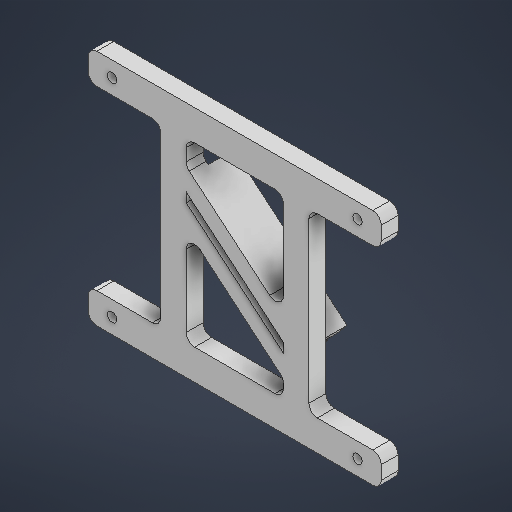
# Autodesk Inventor part: rpi-mount
Saved by Autodesk Inventor 2025 (Build 290162000, 162)
## iProperties
Created: 2024-09-27
Part Number: rpi-mount
Material: Generic
Document SubType Name: Modeling
Designer: Windows 7 was better
Density: 1 g/cm^3
Appearance: Default
Author: Windows 7 was better
Autodesk Inventor part; units mm, degrees
ref_plane "YZ Plane" through (0, 0, 0) normal (1, 0, 0) x (0, 1, 0)
ref_plane "XZ Plane" through (0, 0, 0) normal (0, 1, 0) x (-1, 0, 0)
ref_plane "XY Plane" through (0, 0, 0) normal (0, 0, 1) x (1, 0, 0)
sketch "Sketch1" plane through (0, 0, 0) normal (0, 0, 1) x (1, 0, 0)
  line L0 (35, 0) -> (35, -4)
  line L1 (0, -4) -> (0, 0)
  line L2 (0, 0) -> (0, 1.8) construction
  line L3 (35, 1.8) -> (35, 5.8)
  line L4 (0, 5.8) -> (0, 1.8)
  line L5 (-11.5, 0.9) -> (-11.5, 25.4) construction
  line L6 (-11.5, 25.4) -> (-11.5, -23.6) construction
  line L7 (-11.5, -23.6) -> (46.5, -23.6) construction
  line L8 (-11.5, 25.4) -> (46.5, 25.4) construction
  circle A0 centre (46.5, 25.4) radius 1.1
  circle A1 centre (-11.5, 25.4) radius 1.1
  circle A2 centre (-11.5, -23.6) radius 1.1
  circle A3 centre (46.5, -23.6) radius 1.1
  line L9 (-17.1, -20) -> (52.1, -20)
  line L10 (52.1, -20) -> (52.1, -27.2)
  line L11 (52.1, -27.2) -> (-17.1, -27.2)
  line L12 (-17.1, -27.2) -> (-17.1, -20)
  line L13 (-17.1, -20) -> (52.1, -27.2) construction
  line L14 (52.1, -20) -> (-17.1, -27.2) construction
  line L15 (-17.1, 29) -> (52.1, 29)
  line L16 (52.1, 29) -> (52.1, 21.8)
  line L17 (52.1, 21.8) -> (-17.1, 21.8)
  line L18 (-17.1, 21.8) -> (-17.1, 29)
  line L19 (-17.1, 29) -> (52.1, 21.8) construction
  line L20 (52.1, 29) -> (-17.1, 21.8) construction
  line L21 (35, 21.8) -> (29, 21.8)
  line L22 (29, 21.8) -> (29, -20)
  line L23 (29, -20) -> (35, -20)
  line L24 (35, -20) -> (35, 21.8)
  line L25 (0, 21.8) -> (6, 21.8)
  line L26 (6, 21.8) -> (6, -20)
  line L27 (6, -20) -> (0, -20)
  line L28 (0, -20) -> (0, 21.8)
  line L29 (17.5, 25.4) -> (17.5, 0) construction
  line L30 (17.5, 0) -> (4.0942, 11.2488) construction
  line L31 (4.0942, 11.2488) -> (4.6406, 11.8999) construction
  line L32 (4.6406, 11.8999) -> (3.5479, 10.5976) construction
  line L33 (3.5479, 10.5976) -> (30.3594, -11.8999)
  line L34 (30.3594, -11.8999) -> (27.7883, -14.9641)
  line L35 (27.7883, -14.9641) -> (0.9767, 7.5335)
  line L36 (0.9767, 7.5335) -> (3.5479, 10.5976)
  line L37 (4.6406, 11.8999) -> (31.4521, -10.5976)
  line L38 (31.4521, -10.5976) -> (34.0233, -7.5335)
  line L39 (34.0233, -7.5335) -> (7.2117, 14.9641)
  line L40 (7.2117, 14.9641) -> (4.6406, 11.8999)
  line L41 (27.7883, -14.9641) -> (29, -15.9809)
  line L42 (7.2117, 14.9641) -> (6, 15.9809)
  point P0 (17.5, -23.6)
  point P1 (6, 21.8)
  point P2 (29, 21.8)
  point P3 (0, -20)
  point P4 (35, -20)
  point P5 (29, -3.3184)
  point P6 (6, 13.52)
  point P7 (29, -8.54)
  point P8 (29, -10.7592)
  point P9 (6, 8.54)
  point P10 (6, 10.7592)
  point P11 (29, -13.52)
  point P12 (6, 3.3184)
  dimension "d7" = 24.5
  dimension "d8" = 49
  dimension "d9" = 58
  dimension "d10" = 58
  dimension "d11" = 2.2
  dimension "d12" = 2.2
  dimension "d13" = 2.2
  dimension "d14" = 2.2
  dimension "d15" = 69.2
  dimension "d16" = 7.2
  dimension "d17" = 69.2
  dimension "d18" = 7.2
  dimension "d19" = 6
  dimension "d20" = 6
  dimension "d26" = 17.5
  dimension "d27" = 50
  dimension "d28" = 0.85
  dimension "d29" = 1.7
  dimension "d30" = 35
  dimension "d31" = 4
  dimension "d32" = 4
  constraints: 86 end point, 15 parallel, 9 perpendicular, 9 point on line, 6 horizontal, 6 midpoint, 4 centre point, 4 coincident, 3 vertical
  measures "d7" distance of L5.start L5.end
  measures "d8" distance of L5.end L6.end
  measures "d9" distance of L6.end L7.end
  measures "d10" distance of L5.end L8.end
  measures "d11" diameter of A0
  measures "d12" diameter of A1
  measures "d13" diameter of A2
  measures "d14" diameter of A3
  measures "d15" distance of L10.end L11.end
  measures "d16" distance of L9.end L10.end
  measures "d17" distance of L16.end L17.end
  measures "d18" distance of L15.end L16.end
  measures "d19" distance of L23.end L22.end
  measures "d20" distance of L26.end L27.end
  measures "d26" distance of L29.end L30.end
  measures "d27" angle of L29 L30
  measures "d28" distance of L30.end L31.end
  measures "d29" distance of L31.end L32.end
  measures "d30" distance of L32.end L33.end
  measures "d31" distance of L33.end L34.end
  measures "d32" distance of L38.end L37.end
extrude "Extrusion1" add sketch "Sketch1" along normal blind 4 contours L0 L24 L9 L22 L34 L33 L37 L38 L39 L17 L3 | L9 L10 L11 L12 | L17 L18 L15 L16 | L9 L28 L1 L4 L17 L26 L40 L37 L33 L36 L35 | L41 L34 L22 | L35 L36 L33 L26 | L26 L33 L22 L34 L35 | L22 L33 L34 | L39 L38 L37 L22 | L22 L37 L26 L40 L39 | L42 L40 L26 | L37 L40 L26
extrude "Extrusion2" add sketch "Sketch1" against normal blind 6 contours L35 L36 L33 L26 | L26 L33 L22 L34 L35 | L22 L33 L34 | L39 L38 L37 L22 | L22 L37 L26 L40 L39 | L37 L40 L26
fillet "Fillet1" radius 2 16 edges at (52.1, -27.2, 2) (52.1, -20, 2) (35, -20, 2) (35, 21.8, 2) (52.1, 21.8, 2) (52.1, 29, 2) (-17.1, 29, 2) (-17.1, 21.8, 2) (6, 21.8, 2) (29, 21.8, 2) (0, 21.8, 2) (29, -20, 2) (6, -20, 2) (0, -20, 2) (-17.1, -20, 2) (-17.1, -27.2, 2)
fillet "Fillet2" radius 2 4 edges at (6, 15.9809, 2) (29, -3.3184, 2) (29, -15.9809, 2) (6, 3.3184, 2)
fillet "Fillet3" radius 2 2 edges at (18.0464, 0.6511, -6) (16.9536, -0.6511, -6)
body "Solid1"
